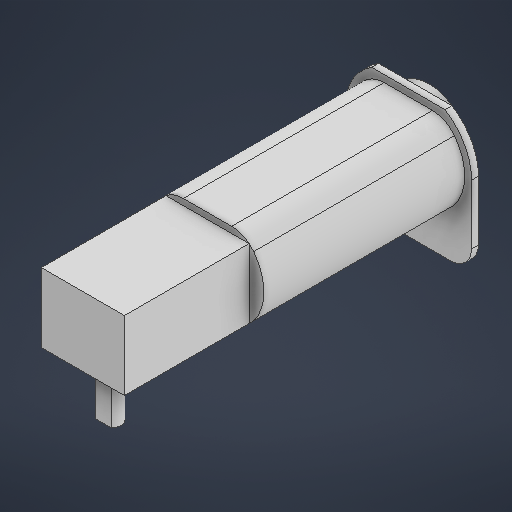
# Autodesk Inventor part: 电机
Saved by Autodesk Inventor 2025 (Build 290162000, 162)
## iProperties
Created: 2025-12-07
Part Number: 电机
Material: 常规
Document SubType Name: Modeling
Designer: XH
Density: 1 g/cm^3
Appearance: 默认
Author: XH
Autodesk Inventor part; units mm, degrees
ref_plane "YZ Plane" through (0, 0, 0) normal (1, 0, 0) x (0, 1, 0)
ref_plane "XZ Plane" through (0, 0, 0) normal (0, 1, 0) x (-1, 0, 0)
ref_plane "XY Plane" through (0, 0, 0) normal (0, 0, 1) x (1, 0, 0)
sketch "草图1" plane through (0, 0, 0) normal (0, 0, 1) x (1, 0, 0)
  line L0 (-5, 0) -> (5, 0) construction
  line L1 (-5, -6.3307) -> (5, -6.3307)
  line L2 (5, 5.4693) -> (-5, 5.4693)
  arc A0 (-5, 5.4693) -> (-5, -6.3307) centre (-1.0059, -0.4307) ccw
  line L3 (0, 0) -> (0, 3.0217)
  arc A1 (5, -6.3307) -> (5, 5.4693) centre (1.0059, -0.4307) ccw
  line L4 (5, 5.4693) -> (5, -6.3307)
  line L5 (-5, 5.4693) -> (-5, -6.3307)
  point P0 (-10.9, 0)
  point P1 (10.9, 0)
  point P2 (10.9, 0)
  dimension "d0" = 11.8
  dimension "d6" = 10
  constraints: 14 end point, 4 point on circle, 2 centre point, 2 perpendicular, 2 symmetric about line, 1 coincident, 1 horizontal, 1 midpoint, 1 parallel, 1 vertical, 1 other
  measures "d0" distance between parallel lines of L1 L2
  measures "d6" distance of L2.start L2.end
extrude "拉伸1" add sketch "草图1" along normal blind 29
sketch "草图2" plane through (0, 0, 29) normal (0, 0, 1) x (1, 0, 0)
  line L0 (6, -5.4307) -> (-6, -5.4307)
  line L1 (-6, -5.4307) -> (-6, 4.5693)
  line L2 (-6, 4.5693) -> (6, 4.5693)
  line L3 (6, 4.5693) -> (6, -5.4307)
  line L4 (6, -5.4307) -> (-6, 4.5693) construction
  line L5 (-6, -5.4307) -> (6, 4.5693) construction
  line L6 (5, 5.4693) -> (-5, 5.4693) projected
  line L7 (0, 5.4693) -> (0, -6.3307)
  line L8 (-5, -6.3307) -> (5, -6.3307) projected
  point P0 (0, -0.4307)
  dimension "d4" = 10
  dimension "d5" = 12
  constraints: 14 end point, 5 midpoint, 2 parallel, 1 horizontal, 1 perpendicular
  measures "d4" distance of L2.end L0.start
  measures "d5" distance between parallel lines of L1 L3
extrude "拉伸2" add sketch "草图2" along normal blind 18
sketch "草图3" plane through (0, 0, 0) normal (0, 0, -1) x (-1, 0, 0)
  line L0 (5, -6.3307) -> (-5, -6.3307) projected
  arc A0 (5, -6.3307) -> (5, 5.4693) centre (1.0059, -0.4307) ccw projected
  line L1 (-5, 5.4693) -> (5, 5.4693) projected
  arc A1 (-5, 5.4693) -> (-5, -6.3307) centre (-1.0059, -0.4307) ccw projected
  arc A2 (5.2957, -7.3307) -> (5.2957, 6.4693) centre (1.0059, -0.4307) ccw
  line L2 (5.2957, -7.3307) -> (-5.2957, -7.3307)
  arc A3 (-5.2957, 6.4693) -> (-5.2957, -7.3307) centre (-1.0059, -0.4307) ccw
  line L3 (-5.2957, 6.4693) -> (5.2957, 6.4693)
  line L4 (-9.1307, -0.4307) -> (9.1307, -0.4307)
  line L5 (9.1307, -0.4307) -> (9.1307, -12.0307)
  line L6 (9.1307, -12.0307) -> (-9.1307, -12.0307)
  line L7 (-9.1307, -12.0307) -> (-9.1307, -0.4307)
  point P0 (0, 0)
  dimension "d9" = 1
  dimension "d10" = 18.5
  constraints: 12 end point, 6 point on circle, 2 centre point, 2 parallel, 1 horizontal, 1 perpendicular, 3 other
  measures "d9" radial gap between concentric circles of A0 A2
  measures "d10" distance between parallel lines of L3 L6
extrude "拉伸3" add sketch "草图3" along normal blind 1
sketch "草图4" plane through (0, 0, -1) normal (0, 0, -1) x (-1, 0, 0)
  circle A0 centre (0, 0) radius 5.5587
  constraints: 1 centre point, 1 coincident
extrude "拉伸4" add sketch "草图4" along normal blind 2
sketch "草图5" plane through (-6, -5.4307, 29) normal (0, 1, 0) x (1, 0, 0)
  circle A0 centre (6, -14) radius 1.5
  line L0 (12, -18) -> (0, -18) projected
  point P0 (6, 29)
  dimension "d15" = 4
  dimension "d16" = 3
  constraints: 1 centre point
  measures "d15" distance from line of A0.centre L0
  measures "d16" diameter of A0
extrude "拉伸5" add sketch "草图5" against normal blind 8
sketch "草图7" plane through (0, -13.4307, 43) normal (0, -1, 0) x (1, 0, 0)
  circle A0 centre (0, 0) radius 1.5 projected
  line L0 (-1.118, 1) -> (1.118, 1)
  point P0 (0, -43)
  point P1 (0, 1.5)
  dimension "d19" = 0.5
  constraints: 3 point on circle, 2 end point, 1 horizontal
  measures "d19" distance edge to line of A0 L0
extrude "拉伸6" cut sketch "草图7" against normal up to surface (8 mm away) contours L0 A0 picked at (-0.0599, 1.1631)
fillet "圆角1" radius 4 4 edges at (-5, 5.4693, 14.5) (5, 5.4693, 14.5) (-5, -6.3307, 14.5) (5, -6.3307, 14.5)
fillet "圆角2" radius 3 2 edges at (-9.1307, -12.0307, -0.5) (9.1307, -12.0307, -0.5)
